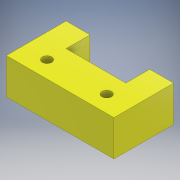
# Autodesk Inventor part: sujetador inferior
Saved by Autodesk Inventor 2018 (Build 220112000, 112)
## iProperties
Created: 2019-05-16
Part Number: sujetador inferior
Material: Generic
Document SubType Name: Modeling
Designer: JLVega003
Density: 1 g/cm^3
Appearance: Yellow
Author: JLVega003
Autodesk Inventor part; units mm, degrees
ref_plane "YZ Plane" through (0, 0, 0) normal (1, 0, 0) x (0, 1, 0)
ref_plane "XZ Plane" through (0, 0, 0) normal (0, 1, 0) x (-1, 0, 0)
ref_plane "XY Plane" through (0, 0, 0) normal (0, 0, 1) x (1, 0, 0)
sketch "Sketch1" plane through (0, 0, 0) normal (0, 0, 1) x (1, 0, 0)
  line L0 (-22.5, 0) -> (22.5, 0)
  line L1 (22.5, 0) -> (22.5, 25)
  line L2 (22.5, 25) -> (12.5, 25)
  line L3 (12.5, 25) -> (12.5, 15)
  line L4 (12.5, 15) -> (-12.5, 15)
  line L5 (-12.5, 15) -> (-12.5, 25)
  line L6 (-12.5, 25) -> (-22.5, 25)
  line L7 (-22.5, 25) -> (-22.5, 0)
  point P0 (0, 0)
  point P1 (0, 0)
  dimension "d0" = 45
  dimension "d1" = 25
  dimension "d2" = 10
  dimension "d3" = 10
  constraints: 16 end point, 6 perpendicular, 2 point on line, 1 coincident, 1 collinear, 1 horizontal, 1 midpoint
  measures "d0" distance between parallel lines of L1 L7
  measures "d1" distance between parallel lines of L2 L0
  measures "d2" distance between parallel lines of L1 L3
  measures "d3" distance between parallel lines of L4 L6
extrude "Extrusion1" add sketch "Sketch1" along normal mid plane 15
sketch "Sketch3" plane through (0, 0, 7.5) normal (0, 0, 1) x (1, 0, 0)
  line L0 (12.5, 7) -> (-12.5, 7) construction
  line L1 (0, 0) -> (0, 14) construction
  line L2 (12.5, 15) -> (-12.5, 15) projected
  point P0 (0, 7)
  dimension "d14" = 8
  dimension "d15" = 25
  constraints: 4 end point, 2 coincident, 2 midpoint, 1 horizontal, 1 perpendicular
  measures "d14" distance between parallel lines of L2 L0
  measures "d15" distance of L0.start L0.end
hole "Hole2" at (12.5, 7, 7.5) at (-12.5, 7, 7.5) direction (0, 0, -1) diameter 4 end through all
body "Solid1"
